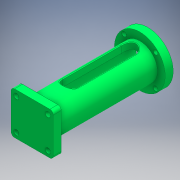
# Autodesk Inventor part: Guida testa a croce
Saved by Autodesk Inventor 2016 (Build 200138000, 138)
## iProperties
Created: 2016-11-29
Part Number: Guida testa a croce
Material: Generic
Document SubType Name: Modeling
Designer: Muhammad
Density: 1 g/cm^3
Appearance: Default
Author: Muhammad
Autodesk Inventor part; units mm, degrees
ref_plane "YZ Plane" through (0, 0, 0) normal (1, 0, 0) x (0, 1, 0)
ref_plane "XZ Plane" through (0, 0, 0) normal (0, 1, 0) x (-1, 0, 0)
ref_plane "XY Plane" through (0, 0, 0) normal (0, 0, 1) x (1, 0, 0)
sketch "Sketch1" plane through (0, 0, 0) normal (0, 1, 0) x (-1, 0, 0)
  line L0 (18.5, 18.5) -> (-18.5, 18.5)
  line L1 (-18.5, 18.5) -> (-18.5, -18.5)
  line L2 (-18.5, -18.5) -> (18.5, -18.5)
  line L3 (18.5, -18.5) -> (18.5, 18.5)
  line L4 (18.5, 18.5) -> (-18.5, -18.5) construction
  line L5 (-18.5, 18.5) -> (18.5, -18.5) construction
  point P0 (0, 0)
  dimension "d0" = 37
  dimension "d1" = 37
  constraints: 12 end point, 2 midpoint, 2 parallel, 1 horizontal, 1 perpendicular
  measures "d0" distance of L2.end L1.end
  measures "d1" distance of L1.end L0.end
extrude "Extrusion1" add sketch "Sketch1" along normal blind 7
sketch "Sketch2" plane through (0, 7, 0) normal (0, 1, 0) x (1, 0, 0)
  circle A0 centre (0, 0) radius 19.5 construction
  line L0 (0, 0) -> (13.7886, 13.7886) construction
  line L1 (0, 0) -> (19.5, 0) construction
  circle A1 centre (13.7886, 13.7886) radius 2.25
  circle A2 centre (-13.7886, 13.7886) radius 2.25
  circle A3 centre (-13.7886, -13.7886) radius 2.25
  circle A4 centre (13.7886, -13.7886) radius 2.25
  dimension "d4" = 39
  dimension "d5" = 45
  dimension "d6" = 4.5
  dimension "d9" = 360
  constraints: 4 centre point, 4 end point, 2 coincident, 1 equal length, 1 horizontal, 12 other
  measures "d5" angle of L1 L0
  measures "d6" diameter of A1
extrude "Extrusion2" cut sketch "Sketch2" against normal through all
fillet "Fillet1" radius 3 4 edges at (-18.5, 3.5, 18.5) (-18.5, 3.5, -18.5) (18.5, 3.5, 18.5) (18.5, 3.5, -18.5)
sketch "Sketch3" plane through (0, 7, 0) normal (0, 1, 0) x (1, 0, 0)
  circle A0 centre (0, 0) radius 15.5
  dimension "d14" = 31
  constraints: 1 centre point, 1 coincident
  measures "d14" diameter of A0
extrude "Extrusion3" add sketch "Sketch3" along normal blind 87.4
sketch "Sketch4" plane through (0, 94.4, 0) normal (0, 1, 0) x (1, 0, 0)
  circle A0 centre (0, 0) radius 10
  dimension "d17" = 20
  constraints: 1 centre point, 1 coincident
  measures "d17" diameter of A0
extrude "Extrusion4" cut sketch "Sketch4" against normal blind 87.4
sketch "Sketch5" plane through (0, 94.4, 0) normal (0, 1, 0) x (1, 0, 0)
  circle A0 centre (0, 0) radius 22.25
  circle A1 centre (0, 0) radius 10
  dimension "d20" = 44.5
  constraints: 2 centre point, 2 coincident
  measures "d20" diameter of A0
extrude "Extrusion5" add sketch "Sketch5" along normal blind 7
sketch "Sketch6" plane through (0, 0, 0) normal (0, 0, 1) x (1, 0, 0)
  line L0 (-10, 101.4) -> (10, 101.4) construction
  line L1 (0, 101.4) -> (0, 90.9) construction
  line L2 (0, 90.9) -> (0, 26.9) construction
  line L3 (0, 90.9) -> (0, 84.4) construction
  line L4 (0, 33.4) -> (0, 84.4) construction
  line L5 (6.5, 33.4) -> (6.5, 84.4)
  line L6 (-6.5, 84.4) -> (-6.5, 33.4)
  arc A0 (-6.5, 33.4) -> (6.5, 33.4) centre (0, 33.4) ccw
  arc A1 (6.5, 84.4) -> (-6.5, 84.4) centre (0, 84.4) ccw
  point P0 (0, 0)
  point P1 (0, 58.9)
  dimension "d23" = 10.5
  dimension "d24" = 64
  dimension "d25" = 6.5
  constraints: 14 end point, 4 point on circle, 4 tangent, 3 midpoint, 2 centre point, 2 vertical, 1 collinear, 1 parallel, 1 point on line
  measures "d23" distance of L1.start L1.end
  measures "d24" distance of L1.end L2.end
  measures "d25" distance of L1.end L3.end
extrude "Extrusion6" cut sketch "Sketch6" along normal through all both and the other way through all
sketch "Sketch7" plane through (0, 101.4, 0) normal (0, 1, 0) x (1, 0, 0)
  circle A0 centre (0, 0) radius 19.5 construction
  circle A1 centre (-13.7886, 13.7886) radius 2.25 construction
  line L0 (0, 0) -> (-13.7886, 13.7886) construction
  circle A2 centre (-13.7886, 13.7886) radius 2
  circle A3 centre (-13.7886, -13.7886) radius 2
  circle A4 centre (13.7886, -13.7886) radius 2
  circle A5 centre (13.7886, 13.7886) radius 2
  dimension "d28" = 39
  dimension "d29" = 4
  dimension "d32" = 360
  constraints: 5 centre point, 2 coincident, 2 end point, 9 other
  measures "d28" diameter of A0
  measures "d29" diameter of A2
extrude "Extrusion7" cut sketch "Sketch7" against normal blind 7
fillet "Fillet2" radius 0.5 9 edges at (-10, 101.4, 0) (0.0434, 90.8999, -15.4999) (0.0434, 90.8999, 15.4999) (6.5, 58.9, -14.0712) (6.5, 58.9, 14.0712) (-0.0002, 26.9, -15.5) (-0.0002, 26.9, 15.5) (-6.5, 58.9, -14.0712) (-6.5, 58.9, 14.0712)
body "Solid1"
